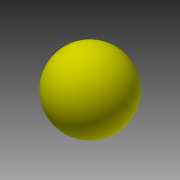
# Autodesk Inventor part: 625-Z_PART3
Saved by Autodesk Inventor 2014 SP2 (Build 180246200, 246)
## iProperties
Created: 2019-11-07
Part Number: 625-Z_PART3
Material: Generic
Catalog Web Link: www.cadenas.de
Description: -Deep groove ball bearings
Vendor: SKF
Document SubType Name: Modeling
Designer: psadmin
Manufacturer: SKF
Mass: 0.00706768 g
Surface Area: 0.178102 cm^2
Volume: 0.00706768 cm^3
Density: 1 g/cm^3
Appearance: PSOLRGB-192-192-192
Category: PARTsolutions
Company: SKF
Title: 625-Z_PART3
Author: Cadenas PARTsolutions
Comments: Deep groove ball bearings
PSOL_IDENT_0: {$CADENAS_DATA\23d-libs\skf\bearings_units_and_housings\ball_bearings\deep_groove_ball_bearings\bb1_
PSOL_IDENT_1: 001_101.prj},189 {VTYP=3D},{NB=625-Z_PART3},{LINA=625-Z_PART3},{NN=BB1_001_101_PART3},{NOPRJ=TRUE},{
PSOL_IDENT_2: DATE=07.11.2019 10:38:24},{GEOMDATE=11.06.2019 11:24:58},{VERSION=},{LINEID=10840},{WBVAR=},{WBNUMER
PSOL_IDENT_3: IC=}  {NB=625-Z_PART3},{LINA=625-Z_PART3},{KT=DUMMY},{PRODUCTID=1050066250},{DESIGNATION=625-Z},{DD=
PSOL_IDENT_4: 5.00},{D=16.000},{B=5.000},{C=0.000},{DD1=8.40},{DD2=0.0},{D1=0.00},{D2=13.22},{D3=0.00},{D4=0.000},
PSOL_IDENT_5: {HH=MIN},{BB=0.000},{FF=0.00},{R0MAX=MIN},{R0=MIN},{R12=0.30},{PITCH=10.20},{DW=2.381},{DDAMIN=7.400
PSOL_IDENT_6: },{DDAMAX=8.300},{DDBMIN=MIN},{DDBMAX=MIN},{DBMIN=MIN},{DAMAX=13.600},{BBAMIN=MIN},{CAMAX=MIN},{RAMA
PSOL_IDENT_7: X=0.300},{LOAD1=1.140},{LOAD2=0.380},{LOAD3=0.016},{SPEED1=95000},{SPEED2=60000},{KR=0.025},{F0=8.40
PSOL_IDENT_8: 0},{Z=8},{II=1},{MASS=0.005},{BEARING=625-Z},{RING=},{HELP=2.102},{HELP2=1.390},{DD1ALG=4.200},{YALG=
PSOL_IDENT_9: 4.200},{PITCH1=10.200},{DW1=2.381},{YALG1=5.898},{HALG1=2.102},{SH=4.200},{CU=0.524},{DESIGN=dgbbz},
PSOL_IDENT_10: {HALG=1.7},{B1=0},{ALGO=1.000}
NT: Deep groove ball bearings
NB: 625-Z_PART3
NBSYN: $DESIGNATION._PART3
LINA: 625-Z_PART3
SUPPLIER: SKF
ARTICLENO: 625-Z_PART3
BOMINFO: 625-Z_PART3
CREATOR: CADENAS GmbH
Autodesk Inventor part; units mm, degrees
ref_plane "YZ Plane" through (0, 0, 0) normal (1, 0, 0) x (0, 1, 0)
ref_plane "XZ Plane" through (0, 0, 0) normal (0, 1, 0) x (-1, 0, 0)
ref_plane "XY Plane" through (0, 0, 0) normal (0, 0, 1) x (1, 0, 0)
sketch "Sketch_6" plane through (0, 0, 0) normal (0, 0, 1) x (1, 0, 0)
  line L0 (3.6905, 5.1) -> (1.3095, 5.1)
  arc A0 (3.6905, 5.1) -> (1.3095, 5.1) centre (2.5, 5.1) ccw
  line L1 (3.6905, 5.1) -> (1.3095, 5.1)
  dimension "d0" = 360
  constraints: 4 end point, 2 point on circle, 1 centre point
revolve "Revolution1" add sketch "Sketch_6" angle 360 about axis through (3.6905, 5.1, 0) along (1, 0, 0)
body "Solid1"
